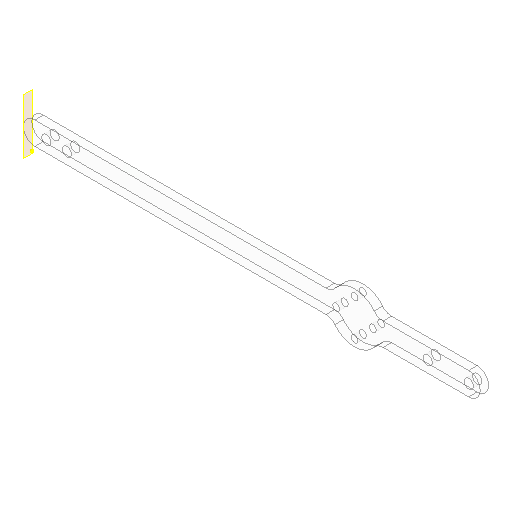
# Autodesk Inventor part: Pendulo
Saved by Autodesk Inventor 2025.3 (Build 293356000, 356)
## iProperties
Created: 2025-11-11
Part Number: Pendulo
Material: PMMA Plastic
Document SubType Name: Modeling
Designer: Gabriel Bojaca
Density: 1.188 g/cm^3
Appearance: Polycarbonate - Clear
Mass: 9.10754 g
Surface Area: 60.1888 cm^2
Volume: 7.66628 cm^3
Author: Gabriel Bojaca
Autodesk Inventor part; units mm, degrees
ref_plane "XZ Plane" through (0, 0, 0) normal (0, 1, 0) x (-1, 0, 0)
ref_plane "XY Plane" through (0, 0, 0) normal (0, 0, 1) x (1, 0, 0)
sketch "Sketch1" plane through (0, 0, 0) normal (0, 0, 1) x (1, 0, 0)
  line L0 (0, 0) -> (200, 0) construction
  line L1 (200, 0) -> (200, 22) construction
  line L2 (200, 22) -> (0, 22) construction
  line L3 (0, 22) -> (0, 0) construction
  line L4 (200, 22) -> (145, 22) construction
  line L5 (145, 22) -> (145, 0) construction
  line L6 (145, 0) -> (200, 0) construction
  line L7 (200, 0) -> (200, 22) construction
  line L8 (200, 11) -> (0, 11) construction
  arc A0 (5, 16) -> (5, 6) centre (5, 11) ccw
  circle A1 centre (10, 11) radius 2
  circle A2 centre (19, 11) radius 2
  arc A3 (195, 6) -> (195, 16) centre (195, 11) ccw
  circle A4 centre (145, 11) radius 8 construction
  circle A5 centre (145, 19) radius 1.5
  circle A6 centre (137, 11) radius 1.5
  circle A7 centre (145, 11) radius 8 construction
  circle A8 centre (145, 3) radius 1.5
  circle A9 centre (153, 11) radius 1.5
  line L9 (132.51, 16) -> (5, 16)
  line L10 (195, 16) -> (157.49, 16)
  line L11 (195, 6) -> (157.49, 6)
  line L12 (132.51, 6) -> (5, 6)
  arc A10 (136.4131, 4.125) -> (153.5869, 4.125) centre (145, 11) ccw
  arc A11 (153.5869, 17.875) -> (136.4131, 17.875) centre (145, 11) ccw
  circle A12 centre (195, 11) radius 2
  circle A13 centre (177, 11) radius 2
  arc A14 (132.51, 16) -> (136.4131, 17.875) centre (132.51, 21) ccw
  arc A15 (136.4131, 4.125) -> (132.51, 6) centre (132.51, 1) ccw
  arc A16 (153.5869, 17.875) -> (157.49, 16) centre (157.49, 21) ccw
  arc A17 (157.49, 6) -> (153.5869, 4.125) centre (157.49, 1) ccw
  point P0 (135.202, 16)
  point P1 (154.798, 6)
  point P2 (135.202, 6)
  point P3 (154.798, 16)
  dimension "d0" = 200
  dimension "d1" = 22
  dimension "d2" = 55
  dimension "d7" = 4
  dimension "d8" = 4
  dimension "d9" = 9
  dimension "d10" = 10
  dimension "d11" = 16
  dimension "d12" = 3
  dimension "d13" = 3
  dimension "d14" = 4
  dimension "d15" = 4
  dimension "d16" = 18
  dimension "d17" = 5
  constraints: 26 end point, 23 point on circle, 17 centre point, 13 tangent, 11 point on line, 8 parallel, 3 equal radius, 3 midpoint, 2 coincident, 2 horizontal, 2 perpendicular, 2 symmetric about line, 1 line through centre, 1 vertical alignment, 4 other
  measures "d0" distance of L2.end L1.end
  measures "d1" distance of L1.end L0.end
  measures "d2" distance of L6.end L5.end
  measures "d7" diameter of A1
  measures "d8" diameter of A2
  measures "d9" distance of A2.centre A1.centre
  measures "d10" distance of point (0, 11) A1.centre
  measures "d11" diameter of A4
  measures "d12" diameter of A5
  measures "d13" diameter of A6
  measures "d14" diameter of A12
  measures "d15" diameter of A13
  measures "d16" distance of A3.centre A13.centre
  measures "d17" radius of A14
extrude "Extrusion1" add sketch "Sketch1" along normal blind 3.7
sketch "Sketch2" plane through (0, 0, 0) normal (1, 0, 0) x (0, 1, 0)
  point P0 (0, 0)
ref_plane "Work Plane1" through (0, 0, 0) normal (1, 0, 0) x (0, 1, 0)
body "Solid1"
